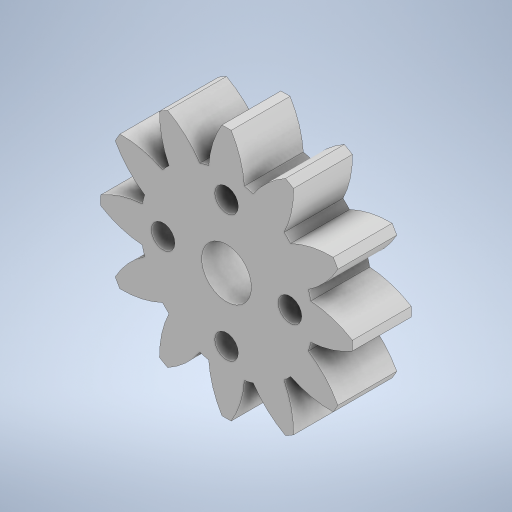
# Autodesk Inventor part: 스텝모터 기어설계
Saved by Autodesk Inventor 2023.1 (Build 271208000, 208)
## iProperties
Created: 2022-08-14
Part Number: 스텝모터 기어설계
Material: 일반
Document SubType Name: Modeling
Designer: fly01
Density: 1 g/cm^3
Appearance: 기본값
Author: fly01
Autodesk Inventor part; units mm, degrees
ref_plane "YZ Plane" through (0, 0, 0) normal (1, 0, 0) x (0, 1, 0)
ref_plane "XZ Plane" through (0, 0, 0) normal (0, 1, 0) x (-1, 0, 0)
ref_plane "XY Plane" through (0, 0, 0) normal (0, 0, 1) x (1, 0, 0)
sketch "스케치1" plane through (0, 0, 0) normal (0, 0, 1) x (1, 0, 0)
  circle A0 centre (0, 0) radius 12 construction
  circle A1 centre (0, 0) radius 14
  circle A2 centre (0, 0) radius 9.5
  line L0 (0, 14.3194) -> (0, 0) construction
  line L1 (-0.57, 15.1413) -> (-0.57, 0.1147) construction
  line L2 (-1.57, 14.5812) -> (-1.57, 0) construction
  line L3 (-2.07, 9.1141) -> (-2.07, 0) construction
  arc A3 (-0.57, 13.9884) -> (-2.07, 9.2717) centre (8.2863, 8.5751) ccw
  arc A4 (2.07, 9.2717) -> (0.57, 13.9884) centre (-8.2863, 8.5751) ccw
  circle A5 centre (0, 0) radius 2.6
  line L4 (-2.5, 1.55) -> (2.5, 1.55)
  line L5 (2.5, 1.55) -> (2.5, -1.55)
  line L6 (2.5, -1.55) -> (-2.5, -1.55)
  line L7 (-2.5, -1.55) -> (-2.5, 1.55)
  line L8 (-2.5, 1.55) -> (2.5, -1.55) construction
  line L9 (2.5, 1.55) -> (-2.5, -1.55) construction
  point P0 (2.0875, 1.55)
  point P1 (2.0875, -1.55)
  point P2 (-2.0875, -1.55)
  point P3 (-2.0875, 1.55)
  point P4 (2.07, 9.2717)
  point P5 (0.57, 13.9884)
  point P6 (-2.5, 0.7141)
  point P7 (-2.5, -0.7141)
  point P8 (2.5, -0.7141)
  point P9 (2.5, 0.7141)
  dimension "d2" = 28
  dimension "d3" = 19
  dimension "d1" = 24
  dimension "d4" = 1.57
  dimension "d5" = 1
  dimension "d6" = 0.5
  dimension "d9" = 5.2
  dimension "d10" = 3.1
  constraints: 20 end point, 5 coincident, 5 parallel, 4 centre point, 4 point on circle, 3 symmetric about line, 2 midpoint, 2 point on line, 1 horizontal, 1 perpendicular, 1 vertical, 7 other
  measures "d1" diameter of A0
  measures "d4" distance between parallel lines of L0 L2
  measures "d5" distance between parallel lines of L1 L2
  measures "d6" distance between parallel lines of L2 L3
  measures "d9" diameter of A5
  measures "d10" distance of L4.end L5.end
extrude "돌출2" add sketch "스케치1" along normal blind 6.5 contours A2 | A5 L5 | L5 A5 L6 L7 L4 | A5 L4 L5 | L5 L6 A5 | L4 A5 | A5 L6 | A5 L7 L4 | L6 L7 A5 | L7 A5
extrude "돌출4" add sketch "스케치1" along normal blind 6.5 contours A4 A2 A3 A1 picked at (-0.4404, 11.4463)
sketch "스케치2" plane through (0, 0, 6.5) normal (0, 0, 1) x (1, 0, 0)
  arc A0 (2.07, 9.2717) -> (-2.07, 9.2717) centre (0, 0) ccw projected
  arc A1 (2.07, 9.2717) -> (0.57, 13.9884) centre (-8.2863, 8.5751) ccw projected
  arc A2 (-2.07, 9.2717) -> (2.07, 9.2717) centre (0, 0) ccw projected
  arc A3 (-1.975, 9.1902) -> (1.975, 9.1902) centre (0, 0) ccw
  arc A4 (1.975, 9.1902) -> (0.5124, 13.8906) centre (-8.2863, 8.5751) ccw
  arc A5 (0.5124, 13.8906) -> (-0.5124, 13.8906) centre (0, 0) ccw
  arc A6 (-0.5124, 13.8906) -> (-1.975, 9.1902) centre (8.2863, 8.5751) ccw
  circle A7 centre (0, 0) radius 9.5
  arc A8 (2.07, 9.2717) -> (0.57, 13.9884) centre (-8.2863, 8.5751) ccw projected
  arc A9 (0.57, 13.9884) -> (-0.57, 13.9884) centre (0, 0) ccw projected
  arc A10 (-0.57, 13.9884) -> (-2.07, 9.2717) centre (8.2863, 8.5751) ccw projected
  point P0 (-1.9682, 9.2939)
  point P1 (1.9682, 9.2939)
  point P2 (2.07, 9.2717)
  point P3 (-1.9682, 9.2939)
  point P4 (-2.07, 9.2717)
  point P5 (1.9682, 9.2939)
  point P6 (0.57, 13.9884)
  point P7 (-2.07, 9.2717)
  constraints: 8 point on circle, 4 centre point, 3 other
extrude "돌출5" cut sketch "스케치2" against normal through all contours A0 A4 A5 A6 A10 A9 A1
pattern_circular "원형 패턴1" count 12 over 360 about axis through (0, 0, 0) along (0, 0, 1) of "돌출5", "돌출4"
sketch "스케치3" plane through (0, 0, 0) normal (0, 0, -1) x (-1, 0, 0)
  circle A0 centre (0, 7) radius 1.3
  circle A1 centre (-7, 0) radius 1.3
  circle A2 centre (0, -7) radius 1.3
  circle A3 centre (7, 0) radius 1.3
  circle A4 centre (0, 0) radius 2.75
  dimension "d23" = 2.6
  dimension "d24" = 7
  dimension "d27" = 360
  dimension "d29" = 5.5
  constraints: 5 centre point, 1 coincident, 9 other
  measures "d23" diameter of A0
  measures "d24" distance of A0.centre point (0, 0)
  measures "d29" diameter of A4
extrude "돌출6" cut sketch "스케치3" against normal through all
